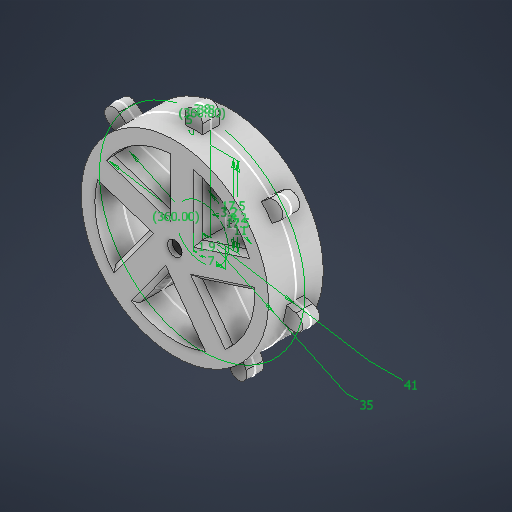
# Autodesk Inventor part: wheel_big
Saved by Autodesk Inventor 2026.2 (Build 302298010, 298A)
## iProperties
Created: 2026-07-08
Part Number: wheel_big
Material: Generic
Document SubType Name: Modeling
Designer: vicke
Density: 1 g/cm^3
Appearance: Default
Author: vicke
Autodesk Inventor part; units mm, degrees
ref_plane "YZ Plane" through (0, 0, 0) normal (1, 0, 0) x (0, 1, 0)
ref_plane "XZ Plane" through (0, 0, 0) normal (0, 1, 0) x (-1, 0, 0)
ref_plane "XY Plane" through (0, 0, 0) normal (0, 0, 1) x (1, 0, 0)
sketch "Sketch1" plane through (0, 0, 0) normal (0, 0, 1) x (1, 0, 0)
  circle A0 centre (0, 0) radius 20.5
  circle A1 centre (0, 0) radius 17.5
  line L0 (-1.9, 17.5) -> (1.9, 17.5)
  line L1 (-1.9, 17.5) -> (-1.9, 22.5)
  line L2 (-1.9, 22.5) -> (1.9, 22.5)
  line L3 (1.9, 22.5) -> (1.9, 17.5)
  circle A2 centre (0, 22.5) radius 1.9
  circle A3 centre (-17.5912, 14.0285) radius 1.9
  line L4 (-16.4066, 15.514) -> (-12.4974, 12.3966)
  line L5 (-18.7758, 12.543) -> (-16.4066, 15.514)
  line L6 (-14.8667, 9.4256) -> (-18.7758, 12.543)
  line L7 (-14.8667, 9.4256) -> (-12.4974, 12.3966)
  circle A4 centre (-21.9359, -5.0067) radius 1.9
  line L8 (-22.3587, -3.1544) -> (-17.484, -2.0418)
  line L9 (-21.5131, -6.8591) -> (-22.3587, -3.1544)
  line L10 (-16.6384, -5.7465) -> (-21.5131, -6.8591)
  line L11 (-16.6384, -5.7465) -> (-17.484, -2.0418)
  circle A5 centre (-9.7624, -20.2718) radius 1.9
  line L12 (-11.4742, -19.4474) -> (-9.3048, -14.9426)
  line L13 (-8.0505, -21.0962) -> (-11.4742, -19.4474)
  line L14 (-5.8811, -16.5913) -> (-8.0505, -21.0962)
  line L15 (-5.8811, -16.5913) -> (-9.3048, -14.9426)
  circle A6 centre (9.7624, -20.2718) radius 1.9
  line L16 (8.0505, -21.0962) -> (5.8811, -16.5913)
  line L17 (11.4742, -19.4474) -> (8.0505, -21.0962)
  line L18 (9.3048, -14.9426) -> (11.4742, -19.4474)
  line L19 (9.3048, -14.9426) -> (5.8811, -16.5913)
  circle A7 centre (21.9359, -5.0067) radius 1.9
  line L20 (21.5131, -6.8591) -> (16.6384, -5.7465)
  line L21 (22.3587, -3.1544) -> (21.5131, -6.8591)
  line L22 (17.484, -2.0418) -> (22.3587, -3.1544)
  line L23 (17.484, -2.0418) -> (16.6384, -5.7465)
  circle A8 centre (17.5912, 14.0285) radius 1.9
  line L24 (18.7758, 12.543) -> (14.8667, 9.4256)
  line L25 (16.4066, 15.514) -> (18.7758, 12.543)
  line L26 (12.4974, 12.3966) -> (16.4066, 15.514)
  line L27 (12.4974, 12.3966) -> (14.8667, 9.4256)
  line L28 (-1.9, 17.5) -> (5.1, 17.5)
  line L29 (5.1, 17.5) -> (5.1, 0)
  line L30 (5.1, 0) -> (-1.9, 0)
  line L31 (-1.9, 0) -> (-1.9, 17.5)
  line L32 (-0.5871, -1.807) -> (-17.2306, 3.6008)
  line L33 (-17.2306, 3.6008) -> (-15.0675, 10.2582)
  line L34 (-15.0675, 10.2582) -> (1.576, 4.8504)
  line L35 (1.576, 4.8504) -> (-0.5871, -1.807)
  line L36 (1.5371, -1.1168) -> (-8.7491, -15.2746)
  line L37 (-8.7491, -15.2746) -> (-14.4122, -11.1601)
  line L38 (-14.4122, -11.1601) -> (-4.126, 2.9977)
  line L39 (-4.126, 2.9977) -> (1.5371, -1.1168)
  line L40 (1.5371, 1.1168) -> (11.8234, -13.041)
  line L41 (11.8234, -13.041) -> (6.1603, -17.1555)
  line L42 (6.1603, -17.1555) -> (-4.126, -2.9977)
  line L43 (-4.126, -2.9977) -> (1.5371, 1.1168)
  line L44 (-0.5871, 1.807) -> (16.0564, 7.2148)
  line L45 (16.0564, 7.2148) -> (18.2195, 0.5574)
  line L46 (18.2195, 0.5574) -> (1.576, -4.8504)
  line L47 (1.576, -4.8504) -> (-0.5871, 1.807)
  point P0 (-17.1432, 11.241)
  point P1 (-20.3228, -2.6897)
  point P2 (-21.5131, -6.8591)
  point P3 (-19.4772, -6.3944)
  point P4 (-10.5682, -17.566)
  point P5 (-7.1445, -19.2147)
  point P6 (7.1445, -19.2147)
  point P7 (10.5682, -17.566)
  point P8 (19.4772, -6.3944)
  point P9 (22.3587, -3.1544)
  point P10 (20.3228, -2.6897)
  point P11 (17.1432, 11.241)
  point P12 (16.4066, 15.514)
  point P13 (14.7739, 14.212)
  point P14 (1.9, 20.4118)
  point P15 (-1.9, 20.4118)
  point P16 (-14.7739, 14.212)
  point P17 (-17.1322, 3.5688)
  point P18 (-6.2743, 0.0409)
  point P19 (-13.9657, -10.5455)
  point P20 (11.7626, -12.9573)
  point P21 (5.052, -3.721)
  point P22 (17.497, 0.3227)
  point P23 (15.958, 7.1828)
  point P24 (5.1, 3.6549)
  point P25 (5.1, 16.7404)
  point P26 (-8.6883, -15.1909)
  point P27 (-1.9777, -5.9546)
  point P28 (5.7138, -16.5409)
  point P29 (-1.9, 17.3966)
  point P30 (-1.9, 5.9798)
  point P31 (-14.3451, 10.0234)
  point P32 (16.4066, 15.514)
  point P33 (22.3587, -3.1544)
  point P34 (11.4742, -19.4474)
  point P35 (-21.5131, -6.8591)
  dimension "d0" = 35
  dimension "d1" = 41
  dimension "d2" = 3.8
  dimension "d4" = 1.9
  dimension "d5" = 17.5
  dimension "d6" = 5
  dimension "d7" = 3.8
  dimension "d11" = 360
  dimension "d13" = 7
  dimension "d14" = 17.5
  dimension "d17" = 360
  constraints: 96 end point, 2 centre point, 2 coincident, 2 horizontal, 2 parallel, 2 perpendicular, 1 midpoint, 1 vertical, 133 other
  measures "d0" diameter of A1
  measures "d1" diameter of A0
  measures "d2" distance of L0.end L0.start
  measures "d4" horizontal distance of point (0, 0) L0.end
  measures "d5" distance from line of point (0, 0) L0
  measures "d6" distance of L0.start L1.end
  measures "d7" distance of L1.end L2.end
  measures "d13" distance between parallel lines of L29 L31
  measures "d14" distance between parallel lines of L0 L30
extrude "Extrusion1" add sketch "Sketch1" along normal mid plane 12 contours A0 L22 L23 A1 L46 L45 L44 L27 L24 | L24 L27 L26 A0 | A0 L20 L23 L22 | L26 L27 A1 L29 L28 L3 A0 | A0 L18 L19 L41 L40 A1 L23 L20 | L3 L0 L1 A0 | A0 L16 L42 L41 L19 L18 | L1 L31 A1 L7 L4 A0 | L28 L29 A1 L0 | L44 L45 A1 | A1 L46 L40 L30 L29 L44 | L29 L44 L35 L34 L31 A1 | A0 L14 L15 A1 L42 L16 | L40 L41 A1 | A1 L42 L36 L47 L46 L40 | L4 L7 L34 L33 L6 A0 | L0 A1 L31 | L45 L46 A1 | L29 L30 L40 L43 L35 L44 | A0 L12 L15 L37 L36 L14 | L42 A1 L19 L16 | L16 L19 L41 L42 | L19 A1 L41 | L46 L47 L36 L39 L30 L40 | L6 L33 L32 A1 L11 L8 A0 | L44 L47 L39 L31 L34 L35 | L35 L47 L44 | A0 L10 L11 A1 L38 L37 L15 L12 | L30 L43 L40 | L8 L11 L10 A0 | L33 L34 L7 L6 | L6 L7 L34 A1 L33 | A1 L34 L7 | L31 L39 L38 L32 A1 L34 | L43 L32 L38 L39 L31 L30 | L47 L36 L42 L43 L32 L35 | L30 L31 L39 | L35 L32 L43 | L39 L36 L47 | L15 L36 A1 | L36 A1 L38 L32 L43 L42 | A1 L32 L33 | L37 A1 L36 L15 | L15 L36 L37 | L37 L38 A1
extrude "Extrusion2" add sketch "Sketch1" along normal mid plane 3.7 contours A0 L22 L23 A1 L46 L45 L44 L27 L24 | L24 L27 L26 A0 | A0 L26 A8 L24 | L22 A7 L20 A0 | A0 L20 L23 L22 | L26 L27 A1 L29 L28 L3 A0 | L25 A8 | A8 L25 | A0 L18 L19 L41 L40 A1 L23 L20 | L21 A7 | A7 L21 | L3 L0 L1 A0 | A0 L1 A2 L3 | L18 A6 L16 A0 | A0 L16 L42 L41 L19 L18 | L1 L31 A1 L7 L4 A0 | A2 L2 | L2 A2 | L28 L29 A1 L0 | L44 L45 A1 | A1 L46 L40 L30 L29 L44 | L29 L44 L35 L34 L31 A1 | A0 L14 L15 A1 L42 L16 | L17 A6 | A6 L17 | L40 L41 A1 | A1 L42 L36 L47 L46 L40 | L4 L7 L34 L33 L6 A0 | A0 L6 A3 L4 | L0 A1 L31 | L45 L46 A1 | L29 L30 L40 L43 L35 L44 | L14 A5 L12 A0 | A0 L12 L15 L37 L36 L14 | L42 A1 L19 L16 | L16 L19 L41 L42 | L19 A1 L41 | L46 L47 L36 L39 L30 L40 | L6 L33 L32 A1 L11 L8 A0 | L5 A3 | A3 L5 | L44 L47 L39 L31 L34 L35 | L35 L47 L44 | A0 L10 L11 A1 L38 L37 L15 L12 | L13 A5 | A5 L13 | L30 L43 L40 | L8 L11 L10 A0 | A0 L10 A4 L8 | L33 L34 L7 L6 | L6 L7 L34 A1 L33 | A1 L34 L7 | L31 L39 L38 L32 A1 L34 | L43 L32 L38 L39 L31 L30 | L47 L36 L42 L43 L32 L35 | L30 L31 L39 | L35 L32 L43 | L39 L36 L47 | L15 L36 A1 | L36 A1 L38 L32 L43 L42 | L9 A4 | A4 L9 | A1 L32 L33 | L37 A1 L36 L15 | L15 L36 L37 | L37 L38 A1
sketch "Sketch2" plane through (0, 0, -6) normal (0, 0, -1) x (-1, 0, 0)
  circle A0 centre (0, 0) radius 1.6
  circle A1 centre (0, 0) radius 5.5
  circle A2 centre (0, 0) radius 4.1
  dimension "d23" = 3.2
  dimension "d24" = 11
  dimension "d59" = 8.2
  constraints: 3 centre point, 3 coincident
  measures "d23" diameter of A0
  measures "d24" diameter of A1
  measures "d59" diameter of A2
extrude "Extrusion3" add sketch "Sketch2" along normal blind 1 contours A0 | A1 | A2
chamfer "Chamfer1" distance 1 angle 45 10 edges at (11.2745, -1.6992, 6) (10.529, 5.4189, 6) (5.1, 10.1976, 6) (-1.9, 11.6882, 6) (-8.1225, 8.0016, 6) (-11.7033, 1.8048, 6) (-10.12, -5.2523, 6) (-5.333, -10.5727, 6) (1.868, -11.2478, 6) (8.4073, -8.3391, 6)
sketch "Sketch4" plane through (0, 0, 6) normal (0, 0, 1) x (1, 0, 0)
  circle A0 centre (0, 0) radius 1.6
  dimension "d60" = 3.2
  constraints: 1 centre point, 1 coincident
  measures "d60" diameter of A0
extrude "Extrusion8" cut sketch "Sketch2" along normal blind 10 and the other way blind 11 contours A2
extrude "Extrusion9" cut sketch "Sketch4" against normal up to surface (13 mm away)
fillet "Fillet2" radius 0.5 1 edges at (4.1, 0, -7)
body "Solid1"
